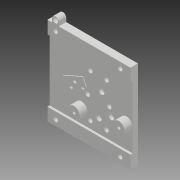
# Autodesk Inventor part: baseplate_gershow
Saved by Autodesk Inventor 2017.3 (Build 213257000, 257)
## iProperties
Created: 2018-06-19
Part Number: baseplate_gershow
Material: Generic
Document SubType Name: Modeling
Designer: Akihiro
Density: 1 g/cm^3
Appearance: Default
Author: Akihiro
Autodesk Inventor part; units mm, degrees
sketch "Sketch1" plane through (0, 0, 0) normal (0, 1, 0) x (-1, 0, 0)
  line L0 (0, 0) -> (98, 0)
  line L1 (98, 0) -> (98, -104)
  line L2 (98, -104) -> (0, -104)
  line L3 (0, -104) -> (0, 0)
  dimension "bplength" = 104
  dimension "bpwidth" = 98
  constraints: 8 end point, 2 parallel, 1 horizontal, 1 perpendicular
  measures "bplength" distance of L2.end L0.start
  measures "bpwidth" distance of L0.start L0.end
extrude "Extrusion1" add sketch "Sketch1" along normal blind 6.35
sketch "cp adapter placement" plane through (0, 0, 0) normal (0, -1, 0) x (1, 0, 0)
  line L0 (-21.8, -15.18) -> (-78.95, -15.18) projected
  arc A0 (-85.1095, -6.925) -> (-91.8405, -6.925) centre (-88.475, -6.925) ccw projected
  arc A1 (-8.9095, -6.925) -> (-15.6405, -6.925) centre (-12.275, -6.925) ccw projected
  arc A2 (-91.8405, -97.015) -> (-85.1095, -97.015) centre (-88.475, -97.015) ccw projected
  line L1 (-85.1095, -88.76) -> (-78.95, -88.76) projected
  line L2 (-78.95, -88.76) -> (-21.8, -88.76) projected
  arc A3 (-15.6405, -97.015) -> (-8.9095, -97.015) centre (-12.275, -97.015) ccw projected
  line L3 (-98, 0) -> (0, 0) projected
  line L4 (0, 0) -> (0, -104) projected
  line L5 (-98, 0) -> (0, 0)
  line L6 (0, 0) -> (0, -15.18)
  line L7 (0, -15.18) -> (-98, -15.18)
  line L8 (-98, -15.18) -> (-98, 0)
  line L9 (-98, -104) -> (0, -104)
  line L10 (0, -104) -> (0, -88.76)
  line L11 (0, -88.76) -> (-98, -88.76)
  line L12 (-98, -88.76) -> (-98, -104)
  line L13 (-98, -104) -> (0, -104) projected
  line L14 (-98, 0) -> (-98, -104) projected
  constraints: 16 end point, 4 collinear, 4 parallel, 2 horizontal, 2 perpendicular, 2 point on line
sketch "grating mount placement" plane through (0, 0, 0) normal (0, -1, 0) x (1, 0, 0)
  circle A0 centre (-67.6981, -48.8255) radius 2.3876 projected
  line L0 (-54.2804, -47.819) -> (-58.0907, -39.0893) projected
  line L1 (-54.2804, -47.819) -> (-77.5596, -57.9798) construction
  line L2 (-77.5596, -57.9798) -> (-81.3698, -49.2501) projected
  line L3 (-81.3698, -49.2501) -> (-58.0907, -39.0893) projected
  circle A1 centre (-67.6981, -48.8255) radius 2.3876 projected
  line L4 (-77.3055, -58.5617) -> (-54.0264, -48.401) projected
  circle A2 centre (-71.9397, -57.8563) radius 1.5
  circle A3 centre (-58.1922, -51.8559) radius 1.5
  line L5 (-57.9305, -71.2041) -> (-65.666, -53.4814) construction
  line L6 (-77.5596, -57.9798) -> (-77.3055, -58.5617)
  line L7 (-54.2804, -47.819) -> (-54.0264, -48.401)
  point P0 (0, 0)
  dimension "d33" = 15
  dimension "d34" = 3
  constraints: 6 end point, 2 centre point, 2 midpoint, 2 tangent, 1 parallel, 1 perpendicular, 1 point on line, 1 other
  measures "d33" distance of A3.centre A2.centre
  measures "d34" diameter of A3
sketch "post mount placement" plane through (0, 0, 0) normal (0, -1, 0) x (1, 0, 0)
  circle A0 centre (-7.4577, -61.8058) radius 6.858 construction
  circle A1 centre (-7.4577, -61.8058) radius 4.445 construction
  circle A2 centre (-7.4577, -61.8058) radius 1.5 construction
  circle A3 centre (-60.3883, -72.8764) radius 6.858 construction
  circle A4 centre (-60.3883, -72.8764) radius 4.445 construction
  circle A5 centre (-60.3883, -72.8764) radius 1.5 construction
  line L0 (0, -104) -> (0, 0) projected
  circle A6 centre (-60.3883, -72.8764) radius 7.1
  circle A7 centre (-7.4577, -61.8058) radius 7.1
  dimension "d7" = 14.2
  constraints: 2 centre point, 2 coincident, 1 equal radius
  measures "d7" diameter of A6
ref_plane "Work Plane1" through (-21.8, -2.54, -103.746) normal (0, 1, 0) x (0, 0, 1)
extrude "CP support" add sketch "cp adapter placement" along normal up to surface (2.54 mm away) contours L0 L7 L8 L3 L4 | L4 L9 L12 L11 L1 L2
ref_plane "Work Plane2" through (-16.1156, -9.05, -70.4636) normal (0, 1, 0) x (0.3125383, 0, 0.9499052)
extrude "post supports" add sketch "post mount placement" along normal up to surface (9.05 mm away)
ref_plane "Work Plane3" through (-81.3698, -0.9112, -57.9798) normal (0, 1, 0) x (-0.4000291, 0, 0.9165024)
extrude "grating support" add sketch "grating mount placement" along normal up to surface (0.9112 mm away) contours A0 | L7 L4 L6 L2 L3 L0
sketch "Sketch5" plane through (-98, -2.54, -88.76) normal (0, -1, 0) x (1, 0, 0)
  point P0 (98, 88.76)
  point P1 (85.725, -8.255)
  point P2 (9.525, -8.255)
  point P3 (9.525, 81.835)
  point P4 (85.725, 81.835)
hole "Hole1" at (-12.275, -2.54, -97.015) at (-88.475, -2.54, -97.015) at (-88.475, -2.54, -6.925) at (-12.275, -2.54, -6.925) direction (0, 1, 0) diameter 5.1308 end through all
sketch "Sketch7" plane through (0, 6.35, 0) normal (0, 1, 0) x (1, 0, 0)
  circle A0 centre (-60.3883, 72.8764) radius 7.1 projected
  circle A1 centre (-7.4577, 61.8058) radius 7.1 projected
  circle A2 centre (-7.4577, 61.8058) radius 7.1 projected
  point P0 (0, 0)
  constraints: 2 coincident
hole "Hole2" at (-60.3883, 6.35, -72.8764) at (-7.4577, 6.35, -61.8058) direction (0, -1, 0) diameter 3.264 end through all counterbore diameter 5.558 counterbore depth 5.08 clearance for "Socket Head Cap Screw" size "#4" standard "Ansi Unified Screw Threads"
sketch "Sketch8" plane through (-77.3055, -0.9112, -58.5617) normal (0, -1, 0) x (0.9165024, 0, 0.4000291)
  point P0 (94.2771, 22.7475)
  point P1 (12.7, 5.08)
hole "Hole3" at (-67.6981, -0.9112, -48.8255) direction (0, 1, 0) diameter 3.429 end through all
sketch "Sketch9" plane through (0, 0, 0) normal (0, -1, 0) x (1, 0, 0)
  circle A0 centre (-71.9397, -57.8563) radius 1.5 projected
  circle A1 centre (-58.1922, -51.8559) radius 1.5 projected
  point P0 (0, 0)
extrude "grating alignment" add sketch "Sketch9" along normal blind 2
sketch "Sketch10" plane through (0, 0, 0) normal (0, -1, 0) x (1, 0, 0)
  circle A0 centre (-39.9322, -72.6284) radius 3.0988 projected
  line L0 (-63.5195, -101.0201) -> (-37.2305, -101.0201) projected
  circle A1 centre (-25.3674, -64.2194) radius 3.0988 projected
  circle A2 centre (-36.7207, -44.0318) radius 3.0988 projected
  point P0 (0, 0)
  constraints: 3 coincident
ref_plane "Work Plane4" through (-52.7377, 3.81, -86.6945) normal (0, 1, 0) x (-0.5, 0, 0.8660254)
extrude "Extrusion6" cut sketch "Sketch10" against normal up to surface (3.81 mm away)
sketch "Sketch11" plane through (-98, -2.54, 0) normal (0, -1, 0) x (1, 0, 0)
  circle A0 centre (9.3758, 4.0988) radius 3.0988 projected
  line L0 (13.4746, 0) -> (5.277, 0)
  line L1 (5.277, 0) -> (5.277, 4.0988)
  line L2 (98, 0) -> (0, 0) projected
  circle A1 centre (9.3758, 4.0988) radius 4.0988 construction
  line L3 (13.4746, 4.0988) -> (13.4746, 0)
  arc A2 (13.4746, 4.0988) -> (5.277, 4.0988) centre (9.3758, 4.0988) ccw
  constraints: 6 end point, 4 point on circle, 3 tangent, 2 centre point, 2 coincident, 1 collinear, 1 horizontal, 1 parallel, 1 perpendicular
ref_plane "Work Plane5" through (-93.0035, 3.81, -0.2805) normal (0, 1, 0) x (0.6799534, 0, 0.7332553)
extrude "Extrusion7" add sketch "Sketch11" against normal up to surface (6.35 mm away)
sketch "Sketch12" plane through (-88.6242, 3.81, 4.0988) normal (0, 1, 0) x (1, 0, 0)
  line L0 (-4.0988, 0) -> (-4.0988, 4.0988) projected
  arc A0 (-4.0988, 0) -> (4.0988, 0) centre (0, 0) ccw projected
  line L1 (4.0988, 4.0988) -> (4.0988, 0) projected
  line L2 (-9.3758, 4.0988) -> (88.6242, 4.0988) projected
extrude "Extrusion8" add sketch "Sketch12" along normal up to surface (2.54 mm away)
sketch "Sketch17" plane through (0, 6.35, 0) normal (0, 1, 0) x (1, 0, 0)
  line L0 (-58.9781, 29.324) -> (-58.9781, 80.124) construction
  circle A0 centre (-67.6981, 48.8255) radius 1.7145 projected
  circle A1 centre (-60.3883, 72.8764) radius 2.779 projected
  circle A2 centre (-7.4577, 61.8058) radius 2.779 projected
  circle A3 centre (-88.475, 6.925) radius 2.5654 projected
  circle A4 centre (-12.275, 97.015) radius 2.5654 projected
  circle A5 centre (-88.475, 97.015) radius 2.5654 projected
  circle A6 centre (-12.275, 6.925) radius 2.5654 projected
  line L1 (-98, 0) -> (-92.723, 0) projected
  line L2 (-92.723, -4.0988) -> (-92.723, 0) projected
  arc A7 (-92.723, -4.0988) -> (-84.5254, -4.0988) centre (-88.6242, -4.0988) ccw projected
  line L3 (-84.5254, 0) -> (-84.5254, -4.0988) projected
  line L4 (-84.5254, 0) -> (0, 0) projected
  line L5 (0, 0) -> (0, 104) projected
  line L6 (0, 104) -> (-98, 104) projected
  line L7 (-98, 104) -> (-98, 0) projected
  circle A8 centre (-27.91, 54.724) radius 3.3655
  circle A9 centre (-53.31, 54.724) radius 3.3655
  arc A10 (-25.3176, 76.7585) -> (-25.3176, 83.4895) centre (-25.3176, 80.124) ccw
  arc A11 (-55.9024, 83.4895) -> (-55.9024, 76.7585) centre (-55.9024, 80.124) ccw
  arc A12 (-25.3176, 25.9585) -> (-25.3176, 32.6895) centre (-25.3176, 29.324) ccw
  arc A13 (-55.9024, 32.6895) -> (-55.9024, 25.9585) centre (-55.9024, 29.324) ccw
  line L8 (-25.3176, 29.324) -> (-55.9024, 29.324) construction
  line L9 (-25.3176, 80.124) -> (-55.9024, 80.124) construction
  line L10 (-40.61, 29.324) -> (-40.61, 80.124) construction
  line L11 (-31.085, 29.231) -> (-31.085, 80.124) construction
  point P0 (-50.135, 80.124)
  point P1 (-50.135, 29.231)
  dimension "d59" = 19.05
  constraints: 10 end point, 8 point on circle, 6 centre point, 3 symmetric about line, 2 coincident, 2 horizontal, 2 midpoint, 1 parallel, 1 perpendicular, 22 other
  measures "d59" distance of point (-50.135, 80.124) L11.end
hole "Hole5" at (-27.91, 6.35, -54.724) at (-53.31, 6.35, -54.724) at (-50.135, 6.35, -80.124) at (-31.085, 6.35, -80.124) at (-31.085, 6.35, -29.231) at (-50.135, 6.35, -29.231) direction (0, -1, 0) diameter 5.1308 end through all
chamfer "top chamfer" distance 0.2 angle 45 33 edges at (-49, -2.54, -15.18) (-98, -2.54, -7.59) (-95.3615, -2.54, 0) (-92.723, -2.54, 2.0494) (-88.6242, -2.54, 8.1976) (-84.5254, -2.54, 2.0494) (-42.2627, -2.54, 0) (0, -2.54, -7.59) (-12.275, -2.54, -4.3596) (-88.475, -2.54, -4.3596) (-50.135, 0, -31.7964) (-31.085, 0, -31.7964) (-39.8195, 0, -44.0318) (-27.91, 0, -57.2894) (-53.31, 0, -57.2894) (-67.6981, -0.9112, -47.111) (-79.3377, -0.9112, -53.9059) (-69.7303, -0.9112, -44.1697) (-56.0585, -0.9112, -43.7452) (-14.5577, -9.05, -61.8058) (-7.4577, -9.05, -63.4378) (-28.4662, 0, -64.2194) (-60.3883, -9.05, -74.5084) (-67.4883, -9.05, -72.8764) (-12.275, -2.54, -94.4496) (-31.085, 0, -82.6894) (-43.031, 0, -72.6284) (-50.135, 0, -82.6894) (-88.475, -2.54, -94.4496) (-98, -2.54, -96.38) (-49, -2.54, -88.76) (-49, -2.54, -104) (0, -2.54, -96.38)
chamfer "Chamfer2" distance 0.2 angle 45 20 edges at (-98, 6.35, -52) (-49, 6.35, -104) (0, 6.35, -52) (-42.2627, 6.35, 0) (-84.5254, 6.35, 2.0494) (-88.6242, 6.35, 8.1976) (-92.723, 6.35, 2.0494) (-88.475, 6.35, -4.3596) (-50.135, 6.35, -31.7964) (-31.085, 6.35, -31.7964) (-12.275, 6.35, -4.3596) (-27.91, 6.35, -57.2894) (-7.4577, 6.35, -64.5848) (-31.085, 6.35, -82.6894) (-12.275, 6.35, -94.4496) (-50.135, 6.35, -82.6894) (-60.3883, 6.35, -75.6554) (-53.31, 6.35, -57.2894) (-67.6981, 6.35, -47.111) (-88.475, 6.35, -94.4496)
equation "\"d51\" = qtrTapProto"
equation "\"d63\" = cham"
equation "\"qtrTapProto\" = 5.1308"
equation "\"cham\" = 0.2"
body "Solid1"
